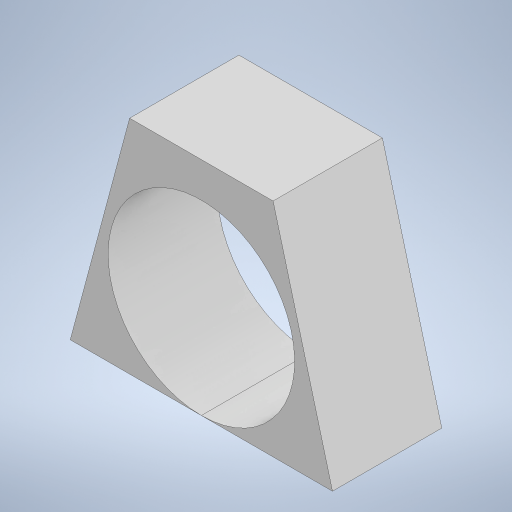
# Autodesk Inventor part: parte ensamble in
Saved by Autodesk Inventor 2024 (Build 280153000, 153)
## iProperties
Created: 2024-03-31
Part Number: parte ensamble in
Material: Generic
Document SubType Name: Modeling
Designer: Admin
Density: 1 g/cm^3
Appearance: Default
Author: Admin
Autodesk Inventor part; units mm, degrees
ref_plane "YZ Plane" through (0, 0, 0) normal (1, 0, 0) x (0, 1, 0)
ref_plane "XZ Plane" through (0, 0, 0) normal (0, 1, 0) x (-1, 0, 0)
ref_plane "XY Plane" through (0, 0, 0) normal (0, 0, 1) x (1, 0, 0)
sketch "Sketch1" plane through (0, 0, 0) normal (0, 0, 1) x (1, 0, 0)
  circle A0 centre (0, 0) radius 8.5375
  line L0 (0, -8.5375) -> (12, -8.5375)
  line L1 (0, -8.5375) -> (-12, -8.5375)
  line L2 (-12, -8.5375) -> (-6.5648, 11.7469)
  line L3 (12, -8.5375) -> (6.5648, 11.7469)
  line L4 (12, -8.5375) -> (33, -8.5375) construction
  line L5 (6.5648, 11.7469) -> (-6.5648, 11.7469)
  dimension "d0" = 17.075
  dimension "d1" = 12
  dimension "d2" = 12
  dimension "d3" = 21
  dimension "d4" = 75
  dimension "d7" = 21
  dimension "d8" = 105
  constraints: 12 end point, 4 horizontal, 1 coincident, 1 equal length, 1 vertical alignment, 2 other
  measures "d1" distance of L0.start L0.end
  measures "d2" distance of L0.start L1.end
  measures "d3" distance of L1.end L2.end
  measures "d4" angle of L1 L2
  measures "d7" distance of L0.end L3.end
  measures "d8" angle of L4 L3
extrude "Extrusion1" add sketch "Sketch1" along normal blind 10
body "Solid1"
